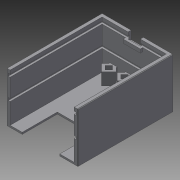
# Autodesk Inventor part: TOP
Saved by Autodesk Inventor 2014 SP1 (Build 180222100, 222)
## iProperties
Created: 2013-12-02
Part Number: TOP
Material: Generic
Document SubType Name: Modeling
Designer: Dominik
Density: 1 g/cm^3
Appearance: Default
Author: Dominik
Autodesk Inventor part; units mm, degrees
ref_plane "YZ Plane" through (0, 0, 0) normal (1, 0, 0) x (0, 1, 0)
ref_plane "XZ Plane" through (0, 0, 0) normal (0, 1, 0) x (-1, 0, 0)
ref_plane "XY Plane" through (0, 0, 0) normal (0, 0, 1) x (1, 0, 0)
sketch "Sketch1" plane through (0, 0, 0) normal (0, 0, 1) x (1, 0, 0)
  line L0 (0, 0) -> (59, 0)
  line L1 (59, 0) -> (59, 79)
  line L2 (59, 79) -> (0, 79)
  line L3 (0, 79) -> (0, 0)
  dimension "d0" = 59
  dimension "d1" = 79
  constraints: 8 end point, 1 horizontal, 1 vertical
  measures "d0" distance between parallel lines of L1 L3
  measures "d1" distance between parallel lines of L2 L0
extrude "Base" add sketch "Sketch1" along normal blind 2
sketch "Sketch2" plane through (0, 0, 2) normal (0, 0, 1) x (1, 0, 0)
  line L0 (59, 0) -> (59, 79) projected
  line L1 (0, 79) -> (0, 0) projected
  line L2 (0, 0) -> (0, 79) projected
  line L3 (0, 79) -> (59, 79) projected
  line L4 (59, 79) -> (59, 0) projected
  line L5 (59, 0) -> (0, 0) projected
  line L6 (3, 0) -> (56, 0)
  line L7 (56, 0) -> (56, 76)
  line L8 (56, 76) -> (3, 76)
  line L9 (3, 76) -> (3, 0)
  dimension "d25" = 3
  dimension "d26" = 3
  dimension "d27" = 3
  constraints: 8 end point, 1 point on line
  measures "d25" distance between parallel lines of L3 L8
  measures "d26" distance between parallel lines of L0 L7
  measures "d27" distance between parallel lines of L1 L9
extrude "Wall" add sketch "Sketch2" along normal blind 39.5 contours L5 L7 L8 L9 L1 L3 L0
sketch "Sketch5" plane through (56, 0, 2) normal (-1, 0, 0) x (0, 0, 1)
  line L0 (39.5, 0) -> (0, 0) projected
  line L1 (0, 76) -> (39.5, 76) projected
  line L2 (0, 76) -> (17, 76) construction
  line L3 (17, 76) -> (17, 0) construction
  line L4 (17, 0) -> (0, 0) construction
  line L5 (0, 0) -> (0, 76) construction
  line L6 (17, 0) -> (19.2, 0)
  line L7 (19.2, 0) -> (19.2, 76)
  line L8 (19.2, 76) -> (17, 76)
  line L9 (17, 76) -> (17, 0)
  point P0 (-2, 0)
  dimension "d28" = 17
  dimension "d29" = 2.2
  constraints: 16 end point, 2 point on line
  measures "d28" distance between parallel lines of L5 L3
  measures "d29" distance between parallel lines of L9 L7
extrude "slider pcb 1" cut sketch "Sketch5" against normal blind 1.5
sketch "Sketch8" plane through (3, 76, 2) normal (0, -1, 0) x (1, 0, 0)
  line L0 (0, 0) -> (0, 39.5) projected
  line L1 (54.5, 19.2) -> (0, 19.2)
  line L2 (0, 19.2) -> (0, 17)
  line L3 (0, 17) -> (54.5, 17)
  line L4 (54.5, 17) -> (54.5, 19.2)
  point P0 (-3, -2)
  constraints: 8 end point, 1 point on line
extrude "slider pcb 2" cut sketch "Sketch8" against normal blind 1.5
sketch "Sketch9" plane through (3, 0, 2) normal (1, 0, 0) x (0, 0, -1)
  line L0 (0, 0) -> (-39.5, 0) projected
  line L1 (-19.2, 77.5) -> (-17, 77.5)
  line L2 (-17, 77.5) -> (-17, 0)
  line L3 (-17, 0) -> (-19.2, 0)
  line L4 (-19.2, 0) -> (-19.2, 77.5)
  point P0 (2, 0)
  constraints: 8 end point, 1 point on line
extrude "slider pcb 3" cut sketch "Sketch9" against normal blind 1.5
sketch "Sketch10" plane through (56, 0, 41.5) normal (-1, 0, 0) x (0, 0, 1)
  line L0 (0, 0) -> (-20.3, 0) projected
  line L1 (-20.3, 76) -> (0, 76) projected
  line L2 (0, 0) -> (-2.9, 0) construction
  line L3 (-2.9, 0) -> (-2.9, 76) construction
  line L4 (-2.9, 76) -> (0, 76) construction
  line L5 (0, 76) -> (0, 0) construction
  line L6 (-2.9, 76) -> (-5.1, 76)
  line L7 (-5.1, 76) -> (-5.1, 0)
  line L8 (-5.1, 0) -> (-2.9, 0)
  line L9 (-2.9, 0) -> (-2.9, 76)
  point P0 (-41.5, 0)
  dimension "d40" = 2.9
  dimension "d41" = 2.2
  constraints: 16 end point, 2 point on line
  measures "d40" distance between parallel lines of L3 L5
  measures "d41" distance between parallel lines of L7 L9
extrude "slider bottom 1" cut sketch "Sketch10" against normal blind 1.5
sketch "Sketch13" plane through (0, 0, 41.5) normal (0, 0, 1) x (1, 0, 0)
  line L0 (3, 76) -> (56, 76) projected
  line L1 (59, 0) -> (59, 79) projected
  line L2 (59, 79) -> (0, 79) projected
  line L3 (0, 79) -> (24.4, 79) construction
  line L4 (24.4, 79) -> (24.4, 76) construction
  line L5 (24.4, 76) -> (0, 76) construction
  line L6 (0, 76) -> (0, 79) construction
  line L7 (34.6, 79) -> (59, 79) construction
  line L8 (59, 79) -> (59, 76) construction
  line L9 (59, 76) -> (34.6, 76) construction
  line L10 (34.6, 76) -> (34.6, 79) construction
  line L11 (24.4, 79) -> (34.6, 79)
  line L12 (34.6, 79) -> (34.6, 76)
  line L13 (34.6, 76) -> (24.4, 76)
  line L14 (24.4, 76) -> (24.4, 79)
  dimension "d48" = 24.4
  dimension "d49" = 24.4
  dimension "d50" = 10.2
  constraints: 24 end point, 3 point on line
  measures "d48" distance between parallel lines of L6 L4
  measures "d49" distance between parallel lines of L1 L10
  measures "d50" distance between parallel lines of L10 L4
extrude "snapper keepout" cut sketch "Sketch13" against normal blind 5.1
sketch "Sketch14" plane through (0, 0, 2) normal (0, 0, 1) x (1, 0, 0)
  line L0 (56, 0) -> (56, 76) projected
  line L1 (3, 76) -> (3, 0) projected
  line L2 (3, 0) -> (56, 0) projected
  line L3 (3, 0) -> (13, 0) construction
  line L4 (13, 0) -> (13, 29) construction
  line L5 (13, 29) -> (3, 29) construction
  line L6 (3, 29) -> (3, 0) construction
  line L7 (13, 29) -> (44, 29)
  line L8 (44, 29) -> (44, 0)
  line L9 (44, 0) -> (13, 0)
  line L10 (13, 0) -> (13, 29)
  point P0 (0, 0)
  dimension "d53" = 29
  dimension "d54" = 10
  dimension "d55" = 12
  constraints: 16 end point, 1 point on line
  measures "d53" distance between parallel lines of L3 L5
  measures "d54" distance between parallel lines of L1 L4
  measures "d55" distance between parallel lines of L0 L8
extrude "led" cut sketch "Sketch14" against normal up to next
chamfer "Chamfer1" distance 0.5 angle 45 16 edges at (46.8, 79, 41.5) (59, 39.5, 41.5) (12.2, 79, 41.5) (0, 39.5, 41.5) (0, 0, 20.75) (6.5, 0, 0) (51.5, 0, 0) (59, 0, 20.75) (59, 39.5, 0) (0, 39.5, 0) (29.5, 79, 0) (59, 79, 20.75) (0, 79, 20.75) (24.4, 79, 38.95) (29.5, 79, 36.4) (34.6, 79, 38.95)
chamfer "Chamfer2" distance 0.5 angle 45 3 edges at (13, 14.75, 0) (28.5, 29, 0) (44, 14.75, 0)
sketch "Sketch15" plane through (3, 76, 21.2) normal (0, -1, 0) x (1, 0, 0)
  line L0 (0, 0) -> (0, 20.3) projected
  line L1 (54.5, 17.4) -> (0, 17.4)
  line L2 (0, 17.4) -> (0, 15.2)
  line L3 (0, 15.2) -> (54.5, 15.2)
  line L4 (54.5, 15.2) -> (54.5, 17.4)
  point P0 (-3, -21.2)
  constraints: 8 end point, 1 point on line
extrude "slider bottom 2" cut sketch "Sketch15" against normal blind 1.5
sketch "Sketch16" plane through (3, 0, 41.5) normal (1, 0, 0) x (0, 0, -1)
  line L0 (20.3, 0) -> (0, 0) projected
  line L1 (5.1, 77.5) -> (2.9, 77.5)
  line L2 (2.9, 77.5) -> (2.9, 0)
  line L3 (2.9, 0) -> (5.1, 0)
  line L4 (5.1, 0) -> (5.1, 77.5)
  point P0 (41.5, 0)
  constraints: 8 end point, 1 point on line
extrude "slider bottom 3" cut sketch "Sketch16" against normal blind 1.5
sketch "Sketch18" plane through (56, 0, 36.4) normal (0, 0, 1) x (1, 0, 0)
  line L0 (-20.9, 79) -> (-32.1, 79) projected
  line L1 (-31.6, 76) -> (-31.6, 78.5) projected
  line L2 (-21.4, 78.5) -> (-21.4, 76) projected
  line L3 (-31.6, 79) -> (-21.4, 79)
  line L4 (-21.4, 79) -> (-21.4, 76)
  line L5 (-21.4, 76) -> (-31.6, 76)
  line L6 (-31.6, 76) -> (-31.6, 79)
  point P0 (-56, 0)
  point P1 (-26.5, 79)
  dimension "d73" = 3
  constraints: 8 end point, 2 point on line, 1 horizontal, 1 midpoint
  measures "d73" distance between parallel lines of L5 L3
extrude "snapper keepout 2" cut sketch "Sketch18" against normal blind 1.7
sketch "Sketch20" plane through (3, 76, 21.2) normal (0, -1, 0) x (1, 0, 0)
  line L0 (53, 15.2) -> (0, 15.2) projected
  line L1 (19.4, 15.2) -> (33.6, 15.2)
  line L2 (33.6, 15.2) -> (33.6, 12.2)
  line L3 (33.6, 12.2) -> (19.4, 12.2)
  line L4 (19.4, 12.2) -> (19.4, 15.2)
  line L5 (31.6, 15.2) -> (31.6, 17.4) projected
  line L6 (21.4, 17.4) -> (21.4, 15.2) projected
  point P0 (-3, -21.2)
  dimension "d79" = 2
  dimension "d80" = 2
  dimension "d81" = 3
  constraints: 8 end point, 1 point on line
  measures "d79" distance between parallel lines of L2 L5
  measures "d80" distance between parallel lines of L4 L6
  measures "d81" distance between parallel lines of L0 L3
extrude "support snapper" add sketch "Sketch20" along normal blind 2
chamfer "Chamfer4" distance 0.5 angle 45 3 edges at (24.4, 79, 35.3) (29.5, 79, 34.7) (34.6, 79, 35.3)
sketch "Sketch3" plane through (0, 0, 0) normal (0, 0, -1) x (-1, 0, 0)
  line L0 (0, 0) -> (-59, 0) projected
  line L1 (0, 79) -> (0, 0) projected
  line L2 (-59, 0) -> (-59, 79) projected
  line L3 (-3, 76) -> (-3, 3) construction
  line L4 (-3, 3) -> (-56, 3) construction
  line L5 (-56, 3) -> (-56, 76) construction
  line L6 (-3, 76) -> (-56, 76) construction
  line L7 (-56, 76) -> (-56, 75) construction
  line L8 (-3, 75) -> (-3, 76) construction
  line L9 (-3, 75) -> (-9.5, 75) construction
  line L10 (-9.5, 75) -> (-9.5, 69) construction
  line L11 (-9.5, 69) -> (-3, 69) construction
  line L12 (-3, 69) -> (-3, 75) construction
  line L13 (-9.5, 69) -> (-15.5, 69) construction
  line L14 (-15.5, 69) -> (-15.5, 75) construction
  line L15 (-15.5, 75) -> (-12.5, 75) construction
  line L16 (-9.5, 75) -> (-9.5, 69) construction
  line L17 (-3, 69) -> (-22.5, 69) construction
  line L18 (-22.5, 69) -> (-22.5, 75) construction
  line L19 (-22.5, 75) -> (-3, 75) construction
  line L20 (-3, 75) -> (-3, 69) construction
  line L21 (-22.5, 69) -> (-28.5, 69) construction
  line L22 (-28.5, 69) -> (-28.5, 75) construction
  line L23 (-22.5, 75) -> (-22.5, 69) construction
  line L24 (-3, 69) -> (-35.5, 69) construction
  line L25 (-35.5, 69) -> (-35.5, 75) construction
  line L26 (-3, 75) -> (-3, 69) construction
  line L27 (-35.5, 69) -> (-41.5, 69) construction
  line L28 (-41.5, 69) -> (-41.5, 75) construction
  line L29 (-35.5, 75) -> (-35.5, 69) construction
  line L30 (-9.5, 69) -> (-15.5, 75) construction
  line L31 (-15.5, 69) -> (-9.5, 75) construction
  line L32 (-22.5, 69) -> (-28.5, 75) construction
  line L33 (-28.5, 69) -> (-22.5, 75) construction
  line L34 (-35.5, 69) -> (-41.5, 75) construction
  line L35 (-41.5, 69) -> (-35.5, 75) construction
  line L36 (-38.5, 66) -> (-44.5, 72)
  line L37 (-35.5, 75) -> (-32.5, 72)
  line L38 (-32.5, 72) -> (-38.5, 66)
  line L39 (-38.5, 66) -> (-38.5, 78) construction
  line L40 (-44.5, 72) -> (-32.5, 72) construction
  line L41 (-25.5, 66) -> (-31.5, 72)
  line L42 (-19.5, 72) -> (-25.5, 66)
  line L43 (-25.5, 66) -> (-25.5, 78) construction
  line L44 (-31.5, 72) -> (-19.5, 72) construction
  line L45 (-12.5, 66) -> (-18.5, 72)
  line L46 (-18.5, 72) -> (-15.5, 75)
  line L47 (-6.5, 72) -> (-12.5, 66)
  line L48 (-12.5, 66) -> (-12.5, 78) construction
  line L49 (-18.5, 72) -> (-6.5, 72) construction
  line L50 (-35.5, 75) -> (-35.5, 76)
  line L51 (-35.5, 76) -> (-41.5, 76)
  line L52 (-41.5, 76) -> (-41.5, 75)
  line L53 (-22.5, 75) -> (-22.5, 76)
  line L54 (-22.5, 76) -> (-28.5, 76)
  line L55 (-28.5, 76) -> (-28.5, 75)
  line L56 (-9.5, 75) -> (-9.5, 76)
  line L57 (-9.5, 76) -> (-15.5, 76)
  line L58 (-15.5, 76) -> (-15.5, 75)
  line L59 (-44.5, 72) -> (-41.5, 75)
  line L60 (-56, 75) -> (-41.5, 75) construction
  line L61 (-31.5, 72) -> (-28.5, 75)
  line L62 (-35.5, 75) -> (-28.5, 75) construction
  line L63 (-35.5, 75) -> (-28.5, 75) construction
  line L64 (-22.5, 75) -> (-3, 75) construction
  line L65 (-22.5, 75) -> (-19.5, 72)
  line L66 (-56, 76) -> (-14.5, 76) construction
  line L67 (-12.5, 76) -> (-3, 76) construction
  line L68 (-22.5, 75) -> (-12.5, 75) construction
  line L69 (-9.5, 75) -> (-3, 75) construction
  line L70 (-9.5, 75) -> (-6.5, 72)
  line L71 (-38.4973, 69.0027) -> (-41.4973, 72.0027)
  line L72 (-41.4973, 72.0027) -> (-38.5027, 74.9973)
  line L73 (-38.5027, 74.9973) -> (-35.5027, 71.9973)
  line L74 (-35.5027, 71.9973) -> (-38.4973, 69.0027)
  line L75 (-38.4973, 69.0027) -> (-38.5027, 74.9973) construction
  line L76 (-41.4973, 72.0027) -> (-35.5027, 71.9973) construction
  line L77 (-25.5, 75) -> (-22.5, 72)
  line L78 (-22.5, 72) -> (-25.5, 69)
  line L79 (-25.5, 69) -> (-28.5, 72)
  line L80 (-28.5, 72) -> (-25.5, 75)
  line L81 (-25.5, 75) -> (-25.5, 69) construction
  line L82 (-22.5, 72) -> (-28.5, 72) construction
  line L83 (-12.5, 69) -> (-15.5, 72)
  line L84 (-15.5, 72) -> (-12.5, 75)
  line L85 (-12.5, 75) -> (-9.5, 72)
  line L86 (-9.5, 72) -> (-12.5, 69)
  line L87 (-12.5, 69) -> (-12.5, 75) construction
  line L88 (-15.5, 72) -> (-9.5, 72) construction
  point P0 (-38.5, 72)
  point P1 (-25.5, 72)
  point P2 (-12.5, 72)
  dimension "d11" = 6.5
  dimension "d12" = 6
  dimension "d13" = 6
  dimension "d14" = 19.5
  dimension "d15" = 6
  dimension "d16" = 32.5
  dimension "d17" = 6
  dimension "d95" = 4.2426
  dimension "d96" = 4.2349
  dimension "d97" = 2.1252
  dimension "d98" = 2.1213
  constraints: 172 end point, 9 horizontal, 9 midpoint, 9 point on line, 5 vertical, 4 parallel, 2 other
  measures "d11" distance between parallel lines of L12 L10
  measures "d12" distance between parallel lines of L9 L11
  measures "d13" distance between parallel lines of L14 L16
  measures "d14" distance between parallel lines of L18 L20
  measures "d15" distance between parallel lines of L22 L23
  measures "d16" distance between parallel lines of L25 L26
  measures "d17" distance between parallel lines of L28 L29
  measures "d95" distance between parallel lines of L74 L72
  measures "d96" distance between parallel lines of L73 L71
  measures "d97" distance between parallel lines of L36 L71
  measures "d98" distance between parallel lines of L41 L79
extrude "Button" add sketch "Sketch3" against normal blind 12
sketch "Sketch22" plane through (0, 0, 2) normal (0, 0, 1) x (1, 0, 0)
  line L0 (28.5, 72) -> (25.5, 75) projected
  line L1 (25.5, 75) -> (22.5, 72) projected
  line L2 (22.5, 72) -> (25.5, 69) projected
  line L3 (25.5, 69) -> (28.5, 72) projected
  line L4 (35.5027, 71.9973) -> (38.4973, 69.0027) projected
  line L5 (38.4973, 69.0027) -> (41.4973, 72.0027) projected
  line L6 (41.4973, 72.0027) -> (38.5027, 74.9973) projected
  line L7 (38.5027, 74.9973) -> (35.5027, 71.9973) projected
  line L8 (9.5, 72) -> (41.4973, 72.0027) construction
  line L9 (12.5, 75) -> (12.5, 69) construction
  line L10 (25.5, 75) -> (25.5, 69) construction
  line L11 (38.5027, 74.9973) -> (38.4973, 69.0027) construction
  circle A0 centre (12.5, 72) radius 2.1213
  circle A1 centre (25.5, 72) radius 2.1213
  circle A2 centre (38.5, 72) radius 2.1213
  point P0 (0, 0)
  constraints: 8 end point, 3 centre point, 3 midpoint
extrude "Extrusion24" cut sketch "Sketch22" against normal up to next contours A1 | A2 L7 L5 | A2 L7 | L5 A2 | A0
chamfer "Chamfer7" distance 0.5 angle 45 3 edges at (36.3787, 72, 0) (23.3787, 72, 0) (10.3787, 72, 0)
equation "\"d26\" = d25"
equation "\"d27\" = d26"
equation "\"d49\" = d48"
body "Solid1"
